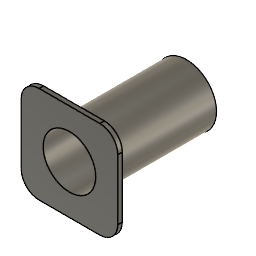
connector to base plate v3 (Autodesk Fusion 360 design; units mm, degrees)
Autodesk Fusion 360 part; units mm, degrees
sketch "Sketch1" plane through (0, 0, 52.25) normal (0, 0, 1) x (-1, 0, 0)
  line L0 (12.25, -100) -> (12.25, 0)
  line L1 (12.25, 0) -> (0, 0)
  line L2 (0, 0) -> (0, -100)
  line L3 (0, -100) -> (12.25, -100)
  line L4 (0, 0) -> (12.25, 0) construction
  line L5 (6.125, 0) -> (8.625, 0) construction
  line L6 (6.125, 0) -> (3.625, 0) construction
  line L7 (3.625, 0) -> (8.625, 0) construction
  line L8 (3.625, 0) -> (8.625, 0)
  line L9 (8.625, 0) -> (8.625, -100)
  line L10 (8.625, -100) -> (3.625, -100)
  line L11 (3.625, -100) -> (3.625, 0)
  dimension "d3" = 5
  constraint coincident L1.end L2.start
  constraint coincident L0.end L1.start
  constraint midpoint L4 L5.start
  constraint horizontal L8
  constraint vertical L9
  constraint horizontal L10
  constraint vertical L11
  constraint coincident L3 L9.end
  measures "d3" distance of L6.end L5.end
extrude "Extrude1" add sketch "Sketch1" along normal blind 5 contours L1 L3 L8 L9 L10 L11
extrude "Extrude2" cut 1 faces at (-5.2917, 66.6667, 57.25) along direction (0, 0, -1) blind 10
sketch "Sketch2" plane through (0, 100, 0) normal (0, 1, 0) x (-1, 0, 0)
  line L0 (-4, 8.6) -> (-4, 3.6)
  line L1 (-4, 3.6) -> (8.5, 3.6)
  line L2 (8.5, 3.6) -> (8.5, 10.6)
  line L3 (8.5, 10.6) -> (3.5, 10.6)
  line L4 (3.5, 10.6) -> (3.5, 8.6)
  line L5 (3.5, 8.6) -> (-4, 8.6)
sketch "Sketch3" plane through (52.1964, 100, 12.1825) normal (0, 1, 0) x (0, 0, -1)
  line L0 (12.1825, 12.1964) -> (8.5825, 12.1964)
  line L1 (8.5825, 12.1964) -> (8.5825, 14.1964)
  line L2 (8.5825, 14.1964) -> (3.5825, 14.1964)
  line L3 (3.5825, 14.1964) -> (3.5825, 12.1964)
  line L4 (3.5825, 12.1964) -> (-0.0675, 12.1964)
  line L5 (-0.0675, 12.1964) -> (-0.0675, 8.5714)
  line L6 (-0.0675, 8.5714) -> (-4.0675, 8.5714)
  line L7 (-4.0675, 8.5714) -> (-4.0675, 3.5714)
  line L8 (-4.0675, 3.5714) -> (-0.0675, 3.5714)
  line L9 (-0.0675, 3.5714) -> (-0.0675, -0.0536)
  line L10 (-0.0675, -0.0536) -> (0.1825, -0.0536)
  line L11 (12.1825, 11.9464) -> (12.1825, 12.1964)
  line L12 (12.1825, 11.9464) -> (-52.2495, 11.9464)
  line L13 (-52.2495, 11.9464) -> (-52.2495, 76.3784)
  line L14 (-52.2495, 76.3784) -> (12.1825, 76.3784)
  line L15 (12.1825, 76.3784) -> (12.1825, 11.9464)
  arc A0 (0.1825, -0.0536) -> (12.1825, 11.9464) centre (0.1825, 11.9464) ccw
  dimension "d8" = 64.432
  dimension "d9" = 64.432
  constraint vertical L13
  constraint perpendicular L12 L13
  constraint horizontal L14
  constraint parallel L13 L15
  constraint coincident L11.start L12.start
  measures "d8" distance of L11.start L12.end
  measures "d9" distance of L11.start L14.end
extrude "Extrude3" add sketch "Sketch3" along normal blind 3 contours L0 L1 L2 L3 L4 L5 L11 L12 L15 | L0 L1 L2 L3 L4 L5 L12 L13 L14 L15
sketch "Sketch4" plane through (0, 103, 0) normal (0, 1, 0) x (-1, 0, 0)
  line L0 (24.182, 0) -> (24.182, 64.432)
  line L1 (24.182, 64.432) -> (-40.25, 64.432)
  line L2 (-40.25, 64.432) -> (-40.25, 0)
  line L3 (-40.25, 0) -> (24.182, 0)
  line L4 (24.182, 64.432) -> (-40.25, 0) construction
  line L5 (24.182, 0) -> (-40.25, 64.432) construction
  circle A0 centre (-8.034, 32.216) radius 17.5
  circle A1 centre (-8.034, 32.216) radius 20
  dimension "d12" = 35
  dimension "d13" = 40
  constraint coincident L0.end L1.start
  constraint coincident L2.end L3.start
  constraint coincident L0.start L3.end
  constraint coincident L1.end L2.start
  constraint midpoint L5 A0.centre
  constraint concentric A0 A1
  measures "d12" diameter of A0
  measures "d13" diameter of A1
extrude "Extrude4" add sketch "Sketch4" along normal blind 75 contours A1
extrude "Extrude5" cut 1 faces at (9.2669, 103, 37.0337) along direction (0, -1, 0) blind 16
move_body "Move1" bodies 1 to x (1, 0, 0) y (0, 1, 0) z (0, 0, 1) at (0, 0, -12)
sketch "Sketch5" plane through (0, 103, 0) normal (0, 1, 0) x (-1, 0, 0)
  line L0 (-40.25, -12) -> (24.182, -12)
  line L1 (24.182, -12) -> (24.182, 52.432)
  line L2 (24.182, 52.432) -> (-40.25, 52.432)
  line L3 (-40.25, 52.432) -> (-40.25, -12)
  circle A0 centre (-8.034, 20.216) radius 20
fillet "Fillet1" radius 12 4 edges at (40.25, 101.5, -12) (40.25, 101.5, 52.432) (-24.182, 101.5, 52.432) (-24.182, 101.5, -12)
